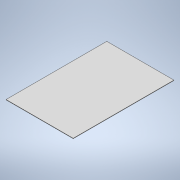
# Autodesk Inventor part: 捨て板
Saved by Autodesk Inventor 2022.3 (Build 263350000, 350)
## iProperties
Created: 2020-12-04
Part Number: 捨て板
Material: Generic
Document SubType Name: Modeling
Designer: masato
Density: 1 g/cm^3
Appearance: Default
Author: Masato Kubotera
Autodesk Inventor part; units mm, degrees
ref_plane "YZ Plane" through (0, 0, 0) normal (1, 0, 0) x (0, 1, 0)
ref_plane "XZ Plane" through (0, 0, 0) normal (0, 1, 0) x (-1, 0, 0)
ref_plane "XY Plane" through (0, 0, 0) normal (0, 0, 1) x (1, 0, 0)
sketch "スケッチ1" plane through (0, 0, 0) normal (0, 0, 1) x (1, 0, 0)
  line L0 (0, 0) -> (200, 0)
  line L1 (200, 0) -> (200, 300)
  line L2 (200, 300) -> (0, 300)
  line L3 (0, 300) -> (0, 0)
  dimension "d4" = 200
  dimension "d5" = 300
  constraints: 8 end point, 2 parallel, 1 coincident, 1 horizontal, 1 perpendicular
  measures "d4" distance of L2.end L1.end
  measures "d5" distance of L1.end L0.end
extrude "押し出し1" add sketch "スケッチ1" against normal blind 1
